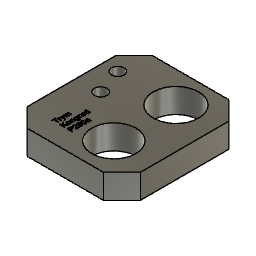
P260a v1_RenngangTool1_byTrymKongrød (Autodesk Fusion 360 design; units mm, degrees)
Autodesk Fusion 360 part; units mm, degrees
note: some values were not read from the file. Set by a fixed rule: which face or edge a step refers to.
sketch "Sketch1" plane through (0, 0, 0) normal (0, 0, 1) x (1, 0, 0)
  line L0 (0, 0) -> (-200, 0)
  line L1 (-200, 0) -> (-200, 200)
  line L2 (-200, 200) -> (0, 200)
  line L3 (0, 200) -> (0, 0)
  dimension "d1" = 200
  dimension "d2" = 200
  constraint horizontal L0
  constraint vertical L1
  constraint horizontal L2
  constraint vertical L3
  constraint coincident L0.start L3.end
  measures "d1" distance of L0.start L0.end
  measures "d2" distance of L0.start L2.end
sketch "Sketch2" plane through (0, 0, 0) normal (0, 0, 1) x (1, 0, 0)
  circle A0 centre (-50, 50) radius 27.25
  dimension "d3" = 54.5
  measures "d3" diameter of A0
sketch "Sketch3" plane through (0, 0, 0) normal (0, 0, 1) x (1, 0, 0)
  circle A0 centre (-50, 126.75) radius 28
  point P0 (-50, 50)
  dimension "d4" = 76.75
  dimension "d5" = 56
  measures "d4" distance of P0 A0.centre
  measures "d5" diameter of A0
sketch "Sketch4" plane through (0, 0, 0) normal (0, 0, 1) x (1, 0, 0)
  circle A0 centre (-121.75, 126.75) radius 7.75
  circle A1 centre (-110.5, 94.25) radius 7.75
  point P0 (-50, 126.75)
  dimension "d6" = 71.75
  dimension "d7" = 15.5
  dimension "d11" = 15.5
  measures "d6" distance of P0 A0.centre
  measures "d7" diameter of A0
  measures "d11" diameter of A1
extrude "Extrude1" add sketch "Sketch2" sketch "Sketch4" sketch "Sketch3" against normal blind 10 of sketch 2 of sketch 3 makes body 1 at (-102.7596, 93.8637, -6.6667) makes body 2 at (-44.3366, 42.8984, 0) makes body 3 at (-114.0096, 126.3637, -6.6667) makes body 4 at (-42.1842, 120.1013, 0)
extrude "Extrude2" add sketch "Sketch1" along normal blind 30 bodies 1 2 3 4
extrude "Extrude3" cut 4 faces at (-42.1842, 120.1013, -10) (-44.3366, 42.8984, -10) (-108.8222, 96.4872, -10) (-121.5569, 128.6484, -10) along direction (0, 0, 1) blind 45 on bodies 1 bodies 1
extrude "Extrude4" cut 1 faces at (-66.6667, 0, 10) along direction (0, 1, 0) blind 10 on bodies 1 bodies 1
extrude "Extrude5" cut 1 faces at (-200, 73.3333, 10) along direction (1, 0, 0) blind 50 on bodies 1 bodies 1
extrude "Extrude6" cut 1 faces at (-100, 200, 10) along direction (0, -1, 0) blind 35 on bodies 1 bodies 1
extrude "Extrude7" cut 1 faces at (-150, 61.6667, 20) along direction (1, 0, 0) blind 10 on bodies 1 bodies 1
chamfer "Chamfer1" distance 23 angle 45 4 edges at (-140, 165, 15) (-140, 10, 15) (0, 10, 15) (0, 165, 15) on bodies 1
sketch "Sketch5" plane through (0, 0, 30) normal (0, 0, 1) x (-1, 0, 0)
  line L0 (0, -142) -> (23, -165)
  line L1 (23, -165) -> (117, -165)
  line L2 (117, -165) -> (140, -142)
  line L3 (140, -142) -> (140, -33)
  line L4 (140, -33) -> (117, -10)
  line L5 (117, -10) -> (23, -10)
  line L6 (23, -10) -> (0, -33)
  line L7 (0, -33) -> (0, -142)
  circle A0 centre (110.5, -94.25) radius 7.75
  circle A1 centre (50, -126.75) radius 28
  circle A2 centre (50, -50) radius 27.25
  circle A3 centre (121.75, -126.75) radius 7.75
  line L8 (92.9693, -33.6034) -> (92.9693, -73.9274) construction
  line L9 (92.9693, -73.9274) -> (110.443, -73.9274) construction
  line L10 (110.443, -73.9274) -> (110.443, -33.6034) construction
  line L11 (110.443, -33.6034) -> (92.9693, -33.6034) construction
  dimension "d27" = 6
  text T0 "Trym Kongrød\nP260a" font "Arial" height 6 align left top in box 40.324 x 17.4737 at (92.9693, -33.6034) x (0, -1) y (1, 0) spacing 1.05 kerned
extrude "Extrude8" cut sketch "Sketch5" against normal blind 2 text T0 bodies 1
